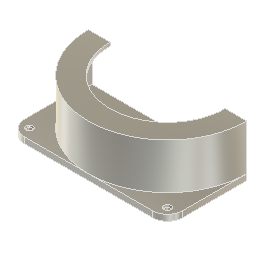
Настенное крепление отрезных дисков для УШМ (Autodesk Fusion 360 design; units mm, degrees)
Autodesk Fusion 360 part; units mm, degrees
sketch "Sketch1" plane through (0, 0, 0) normal (0, 0, 1) x (1, 0, 0)
  line L0 (66, 0) -> (-66, 0)
  arc A0 (-66, 0) -> (66, 0) centre (0, 0) ccw
  arc A1 (-63, 0) -> (63, 0) centre (0, 0) ccw
  line L1 (0, -66) -> (-66, -66)
  line L2 (-66, 0) -> (-66, -66)
  circle A2 centre (-57.5, -57.5) radius 2
  line L3 (0, 1.75) -> (0, 22.5)
  line L4 (66, 0) -> (66, -66)
  circle A3 centre (57.5, -57.5) radius 2
  line L5 (0, -66) -> (66, -66)
  arc A4 (-48, 0) -> (48, 0) centre (0, 0) ccw
  circle A5 centre (-10, -8.5) radius 2
  circle A6 centre (10, -8.5) radius 2
  arc A7 (-35.7911, -20) -> (35.7911, -20) centre (0, 0) ccw
  line L6 (-43.6348, -20) -> (-35.7911, -20)
  line L7 (35.7911, -20) -> (43.6348, -20)
  line L8 (-5, -40.694) -> (-5, -47.7389)
  line L9 (5, -40.694) -> (5, -47.7389)
  dimension "d2" = 126
  dimension "d4" = 4
  dimension "d7" = -15
  dimension "d9" = 4
  dimension "d10" = 4
  dimension "d11" = 8.5
  dimension "d12" = 8.5
  dimension "d13" = 56
  dimension "d14" = 56
  constraint horizontal L0
  constraint concentric A0 A1
  constraint coincident L0 A1.end
  constraint coincident L0 A1.start
  constraint midpoint A0 L1.start
  constraint tangent A0 L1
  constraint horizontal L1
  constraint tangent A0 L2
  constraint perpendicular L1 L2
  constraint symmetric L0.end L3 L0.start
  constraint symmetric L1.start L3 L5.start
  constraint symmetric L1.end L3 L4.end
  constraint symmetric A2 L3 A3
  constraint horizontal L6
  constraint coincident A4 L6.start
  constraint collinear L6 L7
  constraint concentric A4 A7
  constraint coincident A4 L7.end
  constraint coincident A7 L9.start
  constraint coincident A7 L8.start
  constraint coincident A4 L9.end
  constraint coincident A4 L8.end
  measures "d2" diameter of A1
  measures "d4" diameter of A2
  measures "d9" diameter of A5
  measures "d10" diameter of A6
  measures "d11" distance of L0 A5.centre
  measures "d12" distance of L0 A6.centre
  measures "d13" distance of L2 A5.centre
  measures "d14" distance of L4 A6.centre
extrude "Extrude1" add sketch "Sketch1" along normal blind 5 contours L0 A0 A1 | A0 L4 L5 | L0 A1 A4 | A0 L1 L2 | L0 A4 A7 L6 L7 | A4 A7 L8 L9
fillet "Fillet2" radius 3.5 8 edges at (35.7911, -20, 2.5) (43.6348, -20, 2.5) (5, -47.7389, 2.5) (5, -40.694, 2.5) (-43.6348, -20, 2.5) (-35.7911, -20, 2.5) (-5, -40.694, 2.5) (-5, -47.7389, 2.5)
extrude "Extrude2" add sketch "Sketch1" along normal blind 40 contours L0 A0 A1
extrude "Extrude3" add sketch "Sketch1" along normal blind 43 and the other way blind -40 contours L0 A0 A1 | L0 A1 A4
fillet "Fillet1" radius 12.5 2 edges at (-66, -66, 2.5) (66, -66, 2.5)
chamfer "Chamfer1" distance 1 angle 45 4 edges at (-11.8647, -7.7768, 5) (8.1353, -7.7768, 5) (-59.3647, -56.7768, 5) (55.6353, -56.7768, 5)
